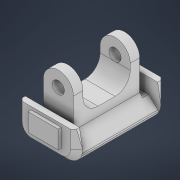
# Autodesk Inventor part: uchytka_spojky_medzi_velkym_strednym
Saved by Autodesk Inventor 2022 (Build 260153000, 153)
## iProperties
Created: 2021-12-17
Part Number: uchytka_spojky_medzi_velkym_strednym
Material: Generic
Document SubType Name: Modeling
Designer: MatusBarany
Density: 1 g/cm^3
Appearance: Default
Author: MatusBarany
Autodesk Inventor part; units mm, degrees
ref_plane "YZ Plane" through (0, 0, 0) normal (1, 0, 0) x (0, 1, 0)
ref_plane "XZ Plane" through (0, 0, 0) normal (0, 1, 0) x (-1, 0, 0)
ref_plane "XY Plane" through (0, 0, 0) normal (0, 0, 1) x (1, 0, 0)
sketch "Sketch2" plane through (0, 0, 0) normal (0, 1, 0) x (-1, 0, 0)
  line L0 (11.1593, 9.222) -> (-8.8407, 9.222)
  line L1 (-8.8407, 9.222) -> (-8.8407, -20.778)
  line L2 (-8.8407, -20.778) -> (11.1593, -20.778)
  line L3 (11.1593, -20.778) -> (11.1593, 9.222)
  point P0 (0, 0)
  dimension "d23" = 30
  dimension "d24" = 20
  constraints: 8 end point, 2 parallel, 1 horizontal, 1 perpendicular
  measures "d23" distance of L0.end L1.end
  measures "d24" distance of L1.end L2.end
extrude "Extrusion2" add sketch "Sketch2" along normal blind 3
sketch "Sketch3" plane through (0, 3, 0) normal (0, 1, 0) x (1, 0, 0)
  line L0 (8.8407, -9.222) -> (8.8407, 20.778) projected
  line L1 (8.8407, 20.778) -> (-11.1593, 20.778) projected
  line L2 (-11.1593, 20.778) -> (-11.1593, -9.222) projected
  line L3 (-11.1593, -9.222) -> (8.8407, -9.222) projected
  line L4 (8.8407, -9.222) -> (8.8407, 20.778) projected
  line L5 (8.8407, 5.778) -> (-11.1593, 5.778)
  line L6 (-11.1593, 20.778) -> (-11.1593, -9.222) projected
  line L7 (8.8407, -7.222) -> (-11.1593, -7.222)
  line L8 (3.8407, -7.222) -> (-6.1593, -7.222)
  line L9 (-6.1593, -7.222) -> (-6.1593, 5.778)
  line L10 (-6.1593, 5.778) -> (3.8407, 5.778)
  line L11 (3.8407, 5.778) -> (3.8407, -7.222)
  line L12 (8.8407, 20.778) -> (8.8407, -9.222)
  line L13 (-11.1593, -9.222) -> (-11.1593, 20.778)
  line L14 (-11.1593, 20.778) -> (8.8407, 20.778)
  line L15 (8.8407, 20.778) -> (8.8407, -9.222)
  line L16 (-11.1593, -9.222) -> (-11.1593, 20.778)
  line L17 (8.8407, 18.778) -> (-11.1593, 18.778)
  line L18 (3.8407, 18.778) -> (-6.1593, 18.778)
  line L19 (-6.1593, 18.778) -> (-6.1593, 5.778)
  line L20 (3.8407, 5.778) -> (3.8407, 18.778)
  point P0 (0, 0)
  point P1 (8.8407, 18.778)
  point P2 (-11.1593, 18.778)
  point P3 (-6.1593, 18.778)
  point P4 (-6.1593, -7.222)
  dimension "d27" = 2
  dimension "d28" = 10
  dimension "d29" = 5
  dimension "d53" = 20
  constraints: 30 end point, 8 symmetric about line, 7 point on line, 2 midpoint, 2 parallel, 2 perpendicular, 1 horizontal
  measures "d27" distance between parallel lines of L3 L7
  measures "d28" distance between parallel lines of L9 L11
  measures "d29" distance between parallel lines of L2 L9
  measures "d53" distance of L13.end L12.start
extrude "Extrusion3" add sketch "Sketch3" along normal blind 3 contours L3 L2 L7 L0 | L7 L9 L5 L11 | L17 L2 L1 L0 | L5 L19 L17 L20
sketch "Sketch4" plane through (0, 6, 0) normal (0, 1, 0) x (1, 0, 0)
  line L0 (8.8407, -7.222) -> (3.8407, -7.222) projected
  line L1 (8.8407, -9.222) -> (8.8407, -7.222) projected
  line L2 (8.8407, -7.222) -> (3.8407, -7.222) projected
  line L3 (3.8407, -7.222) -> (3.8407, 18.778) projected
  line L4 (3.8407, 18.778) -> (8.8407, 18.778) projected
  line L5 (8.8407, 18.778) -> (8.8407, 20.778) projected
  line L6 (8.8407, 20.778) -> (-11.1593, 20.778) projected
  line L7 (-11.1593, 20.778) -> (-11.1593, 18.778) projected
  line L8 (-11.1593, 18.778) -> (-6.1593, 18.778) projected
  line L9 (-6.1593, 18.778) -> (-6.1593, -7.222) projected
  line L10 (-6.1593, -7.222) -> (-11.1593, -7.222) projected
  line L11 (-11.1593, -7.222) -> (-11.1593, -9.222) projected
  line L12 (-11.1593, -9.222) -> (8.8407, -9.222) projected
  line L13 (8.8407, -7.222) -> (-11.1593, -7.222)
  line L14 (8.8407, -9.222) -> (8.8407, 20.778) projected
  line L15 (-11.1593, 18.778) -> (-11.1593, -7.222) projected
  line L16 (-11.1593, 18.778) -> (8.8407, 18.778)
  point P0 (0, 0)
  constraints: 4 end point, 2 perpendicular
extrude "Extrusion4" add sketch "Sketch4" along normal blind 5 contours L1 L12 L11 L10 L13 L0 | L4 L16 L8 L7 L6 L5
ref_plane "Work Plane1" through (8.8407, 0, -5.778) normal (0, 0, -1) x (-1, 0, 0)
chamfer "Chamfer1" distance 1 angle 80 2 edges at (8.8407, 11, 8.222) (-11.1593, 11, 8.222) measured on face at (-10.6593, 11, 8.222) measured on face at (8.3407, 11, 8.222)
chamfer "Chamfer2" distance 1 angle 80 2 edges at (8.8407, 11, -19.778) (-11.1593, 11, -19.778) measured on face at (-10.6593, 11, -19.778) measured on face at (8.3407, 11, -19.778)
sketch "Sketch5" plane through (0, 6, 0) normal (0, 1, 0) x (1, 0, 0)
  line L0 (-6.1593, -7.222) -> (3.8407, -7.222) projected
  line L1 (3.8407, -7.222) -> (3.8407, 18.778) projected
  line L2 (3.8407, 18.778) -> (-6.1593, 18.778) projected
  line L3 (-6.1593, 18.778) -> (-6.1593, -7.222) projected
  line L4 (3.8407, -5.222) -> (-6.1593, -5.222)
  line L5 (-6.1593, 18.778) -> (-6.1593, -7.222) projected
  line L6 (-15.1593, 5.778) -> (12.8407, 5.778) projected
  line L7 (3.8407, 16.778) -> (-6.1593, 16.778)
  point P0 (0, 0)
  point P1 (3.8407, 16.778)
  point P2 (-6.1593, 16.778)
  dimension "d40" = 11
  dimension "d54" = 26
  constraints: 4 end point, 2 point on line, 2 symmetric about line, 1 perpendicular
  measures "d40" distance between parallel lines of L4 L6
  measures "d54" distance of L0.end L1.end
extrude "Extrusion5" add sketch "Sketch5" along normal blind 4 contours L3 L6 L1 L4 | L3 L7 L1 L6
sketch "Sketch6" plane through (0, 10, 0) normal (0, 1, 0) x (1, 0, 0)
  line L0 (-6.1593, -7.222) -> (-6.1593, 18.778) projected
  line L1 (3.8407, 18.778) -> (3.8407, -7.222) projected
  line L2 (3.8407, -5.222) -> (3.8407, -2.0792)
  line L3 (3.8407, -2.0792) -> (-6.1593, -2.0792)
  line L4 (-6.1593, -2.0792) -> (-6.1593, -5.222)
  line L5 (3.8407, 16.778) -> (-6.1593, 16.778) projected
  line L6 (-6.1593, -5.222) -> (3.8407, -5.222) projected
  line L7 (-6.1593, 5.778) -> (3.8407, 5.778)
  line L8 (3.8407, 13.6351) -> (-6.1593, 13.6351)
  point P0 (0, 0)
  point P1 (-6.1593, -2.0792)
  point P2 (-6.1593, 13.6351)
  point P3 (3.8407, 13.6351)
  dimension "d43" = 22
  dimension "d44" = 3.1429
  constraints: 10 end point, 2 midpoint, 2 symmetric about line, 1 parallel, 1 point on line
  measures "d43" distance between parallel lines of L5 L6
  measures "d44" distance between parallel lines of L3 L6
extrude "Extrusion6" add sketch "Sketch6" along normal blind 12 contours L0 L3 L1 L6 | L0 L5 L1 L8
fillet "Fillet1" radius 5 4 edges at (3.8407, 22, 3.6506) (-6.1593, 22, 3.6506) (-6.1593, 22, -15.2065) (3.8407, 22, -15.2065)
fillet "Fillet2" radius 5 2 edges at (-11.1593, 0, -5.778) (8.8407, 0, -5.778)
fillet "Fillet3" radius 5 2 edges at (-1.1593, 10, -13.6351) (-1.1593, 10, 2.0792)
sketch "Sketch9" plane through (-10.1593, 11, 9.222) normal (0, 0, 1) x (1, 0, 0)
  line L0 (0, 0) -> (18, 0) projected
  line L1 (4, -5) -> (4, 6) projected
  line L2 (14, -5) -> (14, 6) projected
  line L3 (0, 0) -> (18, 0) projected
  line L4 (4, 0) -> (14, 0)
  line L5 (14, 0) -> (14, -7)
  line L6 (14, -7) -> (4, -7)
  line L7 (4, -7) -> (4, 0)
  line L8 (4, -1) -> (14, -1)
  point P0 (10.1593, -11)
  point P1 (14, -1)
  point P2 (4, -1)
  dimension "d58" = 6
  dimension "d59" = 1
  dimension "d62" = 10
  constraints: 10 end point, 5 point on line, 2 parallel, 2 perpendicular, 1 horizontal
  measures "d58" distance between parallel lines of L8 L6
  measures "d59" distance between parallel lines of L0 L8
  measures "d62" distance of L8.start L8.end
extrude "Extrusion8" add sketch "Sketch9" along normal blind 1 contours L8 L2 L5 L6 L7 L1
sketch "Sketch10" plane through (-6.1593, 6, 5.222) normal (0, 0, 1) x (1, 0, 0)
  circle A0 centre (5, 11) radius 2
  arc A1 (10, 11) -> (0, 11) centre (5, 11) ccw projected
  point P0 (6.1593, -6)
  dimension "d63" = 4
  constraints: 1 centre point, 1 concentric
  measures "d63" diameter of A0
extrude "Extrusion9" cut sketch "Sketch10" against normal through all
chamfer "Chamfer3" distance 2 angle 45 10 edges at (-1.1593, 0, 9.222) (7.3762, 1.4645, 9.222) (8.8407, 5.1644, 9.222) (-9.6948, 1.4645, 9.222) (-11.1593, 5.1644, 9.222) (-1.1593, 0, -20.778) (-9.6948, 1.4645, -20.778) (-11.1593, 5.1644, -20.778) (7.3762, 1.4645, -20.778) (8.8407, 5.1644, -20.778)
chamfer "Chamfer4" distance 4 angle 45 2 edges at (-6.1593, 3, -5.778) (3.8407, 3, -5.778)
equation "\"d27\" = 0.1 * d53"
equation "\"d28\" = 0.5 * d53"
equation "\"d29\" = 0.25 * d53"
equation "\"d44\" = 0.142857 * d43"
body "Solid2"
